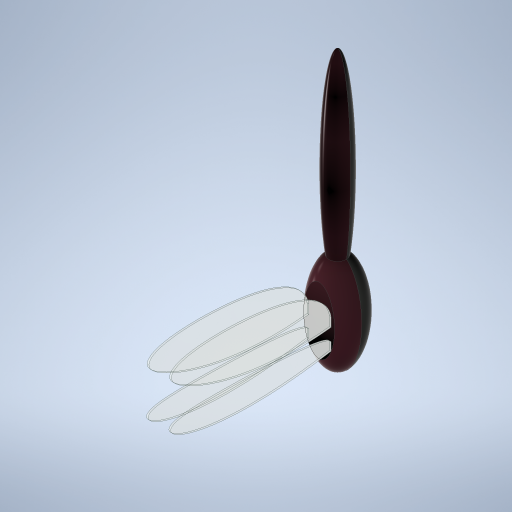
# Autodesk Inventor part: dragonfly
Saved by Autodesk Inventor 2024 (Build 280153000, 153)
## iProperties
Created: 2023-06-15
Part Number: dragonfly
Material: Generic
Document SubType Name: Modeling
Designer: dsdan
Density: 1 g/cm^3
Appearance: Default
Author: dsdan
Autodesk Inventor part; units mm, degrees
ref_plane "XY Plane" through (0, 0, 0) normal (0, 0, 1) x (1, 0, 0)
sketch "Sketch1" plane through (0, 0, 0) normal (0, 1, 0) x (-1, 0, 0)
  arc A0 (2.75, 0) -> (-2.75, 0) centre (0, 0) ccw
  line L0 (2.75, 0) -> (-2.75, 0)
  dimension "d0" = 5.5
  constraints: 2 end point, 2 point on circle, 1 centre point, 1 coincident, 1 horizontal, 1 midpoint
  measures "d0" diameter of A0
revolve "Revolution1" add sketch "Sketch1" angle 360 about axis through (-2.75, 0, 0) along (1, 0, 0)
sketch "Sketch2" plane through (0, 0, 0) normal (0, 0, 1) x (1, 0, 0)
  ellipse E0 centre (0, 8.5905) end of major axis (0, 2.5905) minor radius 2.8
  line L0 (0, 0) -> (0, 35.842)
  ellipse E1 centre (0, 22.8531) end of major axis (0, 10.8531) minor radius 1.5
  point P0 (1.0348, 14.1657)
  point P1 (0, 34.8531)
  point P2 (0, 2.5905)
  dimension "d2" = 6
  dimension "d3" = 12
  dimension "d4" = 2.8
  dimension "d5" = 1.5
  constraints: 2 end point, 2 point on line, 1 vertical, 4 other
revolve "Revolution2" add sketch "Sketch2" angle 360 about axis through (0, 0, 0) along (0, 1, 0) separate body picked at (0.8015, 6.3198) picked at (0.2487, 12.629) picked at (0.4847, 25.0823) contours L0 E1 E0 | E1 L0 E0 | E0 L0 E1
ref_plane "Work Plane1" through (0, 2.75, 0) normal (0, 1, 0) x (-1, 0, 0)
sketch "Sketch4" plane through (0, 2.75, 0) normal (0, 1, 0) x (-1, 0, 0)
  line L0 (4.3908, 4.5491) -> (-4.255, 4.5491)
  line L1 (-4.255, 4.5491) -> (-4.255, 2.15)
  line L2 (-4.255, 2.15) -> (4.3908, 2.15)
  line L3 (4.3908, 2.15) -> (4.3908, 4.5491)
  point P0 (0, 0)
  dimension "d7" = 2.15
  constraints: 8 end point, 2 parallel, 1 horizontal, 1 perpendicular
  measures "d7" distance from line of point (0, 0) L2
extrude "Extrusion1" cut sketch "Sketch4" along normal through all bodies 1 2
ref_plane "Work Plane2" through (0, 0.1, 0) normal (0, 1, 0) x (-1, 0, 0)
sketch "Sketch5" plane through (0, 0.1, 0) normal (0, 1, 0) x (-1, 0, 0)
  circle A0 centre (-1.1, 0.6) radius 2.5
  line L0 (-1.1, 3.1) -> (-1.1, -1.9)
  point P0 (0, 0)
  point P1 (-1.1, 0.6)
  dimension "d11" = 1.1
  dimension "d12" = 5
  dimension "d13" = 0.6
  constraints: 2 end point, 2 point on circle, 1 centre point, 1 midpoint, 1 vertical
  measures "d11" horizontal distance of point (0, 0) A0.centre
  measures "d12" diameter of A0
  measures "d13" vertical distance of point (0, 0) point (-1.1, 0.6)
revolve "Revolution3" add sketch "Sketch5" angle 360 about axis through (1.1, 0.1, 3.1) along (0, 0, -1) picked at (-1.4873, -0.1379) bodies 1 contours L0 A0
mirror "Mirror1" about plane through (0, 0, 0) normal (1, 0, 0) of "Revolution3" bodies 1
ref_plane "Work Plane3" through (1.3, 0, 0) normal (1, 0, 0) x (0, 1, 0)
sketch "Sketch6" plane through (1.3, 0, 0) normal (1, 0, 0) x (0, 1, 0)
  line L0 (4.7468, 2.15) -> (12.4342, 2.15) projected
  line L1 (6.1929, 2.15) -> (4.7468, 10.7237) construction
  line L2 (4.7468, 10.7237) -> (5.9482, 21.443) construction
  line L3 (5.9482, 21.443) -> (8.627, 21.737) construction
  line L4 (8.627, 21.737) -> (8.5526, 18.4086) construction
  line L5 (8.5526, 18.4086) -> (8.2013, 2.6925) construction
  line L6 (8.2013, 2.6925) -> (7.1557, 2.15) construction
  spline S0 degree 4 poles (6.1929, 2.15) (4.7468, 10.7237) (5.9482, 21.443) (8.627, 21.737) (8.5526, 18.4086) (8.2013, 2.6925) (7.1557, 2.15) knots 1 1 1 1 1 2 3 4 4 4 4 4
  line L7 (8.5905, 2.15) -> (7.6487, 10.548) construction
  line L8 (7.6487, 10.548) -> (11.4484, 21.2949) construction
  line L9 (11.4484, 21.2949) -> (13.1845, 21.5889) construction
  line L10 (13.1845, 21.5889) -> (15.1646, 18.656) construction
  line L11 (15.1646, 18.656) -> (13.7782, 2.8512) construction
  line L12 (13.7782, 2.8512) -> (9.674, 2.15) construction
  spline S1 degree 4 poles (8.5905, 2.15) (7.6487, 10.548) (11.4484, 21.2949) (13.1845, 21.5889) (15.1646, 18.656) (13.7782, 2.8512) (9.674, 2.15) knots 1 1 1 1 1 2 3 4 4 4 4 4
  point P0 (0, 0)
  point P1 (9.2566, 2.4465)
  constraints: 3 point on line, 2 midpoint, 6 other
extrude "Extrusion2" add sketch "Sketch6" along normal mid plane 0.2 separate body
mirror "Mirror2" about plane through (0, 0, 0) normal (1, 0, 0) bodies 3
